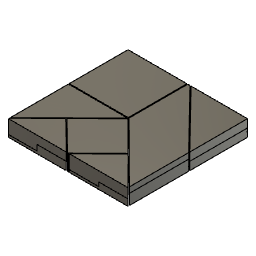
3D Puzzle Pieces v8 (Autodesk Fusion 360 design; units mm, degrees)
Autodesk Fusion 360 part; units mm, degrees
box "BoxPrimitive1" add length 300 width 300 height 18 placed x (0, 0, -1) y (-1, 0, 0) z (0, 1, 0) at (300, 0, 0) makes body 1 in component "CNC Safe Box v6"
sketch "Sketch3" plane through (0, 0, 0) normal (0, 0, 1) x (1, 0, 0) in component "CNC Safe Box v6"
  line L0 (0, 18) -> (0, 0)
  line L1 (0, 0) -> (300, 0)
  line L2 (300, 0) -> (300, 18)
  line L3 (300, 18) -> (0, 18)
  line L4 (42.8571, 18) -> (85.7143, 18)
  line L5 (85.7143, 18) -> (85.7143, 0)
  line L6 (85.7143, 0) -> (42.8571, 0)
  line L7 (42.8571, 0) -> (42.8571, 18)
  dimension "d20" = 42.8571
  dimension "d21" = 18
  dimension "d22" = 42.8571
  constraint horizontal L4
  constraint vertical L5
  constraint horizontal L6
  constraint vertical L7
  constraint coincident L3 L4.start
  measures "d20" distance of L4.start L4.end
  measures "d21" distance of L4.start L6.end
  measures "d22" distance of L0.start L4.start
extrude "Extrude1" cut sketch "Sketch3" against normal blind 18 contours L1 L3 L4 L5 L6 L7 bodies 1 in component "CNC Safe Box v6"
pattern_linear "R-Pattern1" count 3 spacing 85.7143 along (1, 0, 0) of 3 faces at (42.8571, 6, -6) (57.1429, 12, -18) (85.7143, 12, -6) on bodies 1 in component "CNC Safe Box v6"
sketch "Sketch4" plane through (0, 0, 0) normal (-1, 0, 0) x (0, 0, 1) in component "CNC Safe Box v6"
  line L0 (-300, 18) -> (-300, 0)
  line L1 (-300, 0) -> (0, 0)
  line L2 (0, 0) -> (0, 18)
  line L3 (0, 18) -> (-300, 18)
  line L4 (-42.8571, 18) -> (-85.7143, 18)
  line L5 (-85.7143, 18) -> (-85.7143, 0)
  line L6 (-85.7143, 0) -> (-42.8571, 0)
  line L7 (-42.8571, 0) -> (-42.8571, 18)
  dimension "d29" = 42.8571
  dimension "d30" = 18
  dimension "d31" = 42.8571
  constraint horizontal L4
  constraint vertical L5
  constraint horizontal L6
  constraint vertical L7
  constraint coincident L3 L4.start
  measures "d29" distance of L4.start L4.end
  measures "d30" distance of L4.start L6.end
  measures "d31" distance of L2.end L4.start
extrude "Extrude2" cut sketch "Sketch4" against normal blind 18 contours L1 L3 L4 L5 L6 L7 bodies 1 in component "CNC Safe Box v6"
pattern_linear "R-Pattern2" count 3 spacing 85.7143 along (0, 0, -1) of 3 faces at (6, 6, -42.8571) (18, 12, -71.4286) (6, 12, -85.7143) on bodies 1 in component "CNC Safe Box v6"
sketch "Sketch5" plane through (0, 0, 0) normal (0, 0, 1) x (1, 0, 0) in component "CNC Safe Box v6"
  line L0 (0, 0) -> (300, 0)
  line L1 (300, 0) -> (300, 300)
  line L2 (300, 300) -> (0, 300)
  line L3 (0, 300) -> (0, 0)
  dimension "d38" = 300
  dimension "d39" = 300
  constraint horizontal L0
  constraint vertical L1
  constraint horizontal L2
  constraint vertical L3
  constraint coincident L0.start L3.end
  measures "d38" distance of L0.start L0.end
  measures "d39" distance of L0.start L2.end
extrude "Extrude3" add sketch "Sketch5" against normal blind 18 separate body makes body 2 in component "CNC Safe Box v6"
combine "Combine1" operation cut target body 2 tool bodies 1 keep tools in component "CNC Safe Box v6"
sketch "Sketch6" plane through (0, 0, 0) normal (-1, 0, 0) x (0, 0, 1) in component "CNC Safe Box v6"
  line L0 (-18, 18) -> (0, 18)
  line L1 (0, 18) -> (0, 300)
  line L2 (0, 300) -> (-18, 300)
  line L3 (-18, 300) -> (-18, 18)
  line L4 (-18, 60.8571) -> (0, 60.8571)
  line L5 (0, 60.8571) -> (0, 103.7143)
  line L6 (0, 103.7143) -> (-18, 103.7143)
  line L7 (-18, 103.7143) -> (-18, 60.8571)
  dimension "d42" = 18
  dimension "d43" = 42.8571
  dimension "d44" = 42.8571
  constraint horizontal L4
  constraint vertical L5
  constraint horizontal L6
  constraint vertical L7
  constraint coincident L3 L4.start
  measures "d42" distance of L4.start L4.end
  measures "d43" distance of L4.start L6.end
  measures "d44" distance of L0.start L4.start
extrude "Extrude4" cut sketch "Sketch6" against normal blind 18 contours L1 L3 L4 L5 L6 L7 bodies 2 in component "CNC Safe Box v6"
pattern_linear "R-Pattern3" count 3 spacing 85.7143 along (0, 1, 0) of 3 faces at (6, 60.8571, -12) (18, 89.4286, -12) (6, 103.7143, -6) on bodies 2 in component "CNC Safe Box v6"
sketch "Sketch7" plane through (0, 0, 0) normal (1, 0, 0) x (0, 0, -1) in component "CNC Safe Box v6"
  line L0 (0, 0) -> (300, 0)
  line L1 (300, 0) -> (300, 300)
  line L2 (300, 300) -> (0, 300)
  line L3 (0, 300) -> (0, 0)
  dimension "d54" = 300
  dimension "d55" = 300
  constraint horizontal L0
  constraint vertical L1
  constraint horizontal L2
  constraint vertical L3
  constraint coincident L0.start L3.end
  measures "d54" distance of L0.start L0.end
  measures "d55" distance of L0.start L2.end
extrude "Extrude6" add sketch "Sketch7" along normal blind 18 separate body makes body 3 in component "CNC Safe Box v6"
combine "Combine3" operation cut target body 3 tool bodies 2 1 keep tools in component "CNC Safe Box v6"
extrude "Extrude7" add 1 faces at (18, 169.1429, -163.1429) along direction (-1, 0, 0) blind 18 from surface at -282 separate body on bodies 3 makes body 4 in component "CNC Safe Box v6"
combine "Combine4" operation cut target body 1 tool bodies 4 keep tools in component "CNC Safe Box v6"
combine "Combine5" operation cut target body 2 tool bodies 4 keep tools in component "CNC Safe Box v6"
sketch "Sketch8" plane through (0, 0, 0) normal (0, 0, 1) x (1, 0, 0) in component "CNC Safe Box v6"
  line L0 (282, 275.1429) -> (300, 275.1429)
  line L1 (300, 275.1429) -> (300, 300)
  line L2 (300, 300) -> (0, 300)
  line L3 (0, 300) -> (0, 275.1429)
  line L4 (0, 275.1429) -> (18, 275.1429)
  line L5 (18, 275.1429) -> (18, 232.2857)
  line L6 (18, 232.2857) -> (0, 232.2857)
  line L7 (0, 232.2857) -> (0, 189.4286)
  line L8 (0, 189.4286) -> (18, 189.4286)
  line L9 (18, 189.4286) -> (18, 146.5714)
  line L10 (18, 146.5714) -> (0, 146.5714)
  line L11 (0, 146.5714) -> (0, 103.7143)
  line L12 (0, 103.7143) -> (18, 103.7143)
  line L13 (18, 103.7143) -> (18, 60.8571)
  line L14 (18, 60.8571) -> (0, 60.8571)
  line L15 (0, 60.8571) -> (0, 18)
  line L16 (0, 18) -> (42.8571, 18)
  line L17 (42.8571, 18) -> (42.8571, 0)
  line L18 (42.8571, 0) -> (85.7143, 0)
  line L19 (85.7143, 0) -> (85.7143, 18)
  line L20 (85.7143, 18) -> (128.5714, 18)
  line L21 (128.5714, 18) -> (128.5714, 0)
  line L22 (128.5714, 0) -> (171.4286, 0)
  line L23 (171.4286, 0) -> (171.4286, 18)
  line L24 (171.4286, 18) -> (214.2857, 18)
  line L25 (214.2857, 18) -> (214.2857, 0)
  line L26 (214.2857, 0) -> (257.1429, 0)
  line L27 (257.1429, 0) -> (257.1429, 18)
  line L28 (257.1429, 18) -> (300, 18)
  line L29 (300, 18) -> (300, 60.8571)
  line L30 (300, 60.8571) -> (282, 60.8571)
  line L31 (282, 60.8571) -> (282, 103.7143)
  line L32 (282, 103.7143) -> (300, 103.7143)
  line L33 (300, 103.7143) -> (300, 146.5714)
  line L34 (300, 146.5714) -> (282, 146.5714)
  line L35 (282, 146.5714) -> (282, 189.4286)
  line L36 (282, 189.4286) -> (300, 189.4286)
  line L37 (300, 189.4286) -> (300, 232.2857)
  line L38 (300, 232.2857) -> (282, 232.2857)
  line L39 (282, 232.2857) -> (282, 275.1429)
  circle A0 centre (269, 300) radius 13
  line L40 (300, 300) -> (240, 300)
  line L41 (240, 300) -> (240, 320)
  line L42 (240, 320) -> (300, 320)
  line L43 (300, 320) -> (300, 300)
  dimension "d61" = 26
  dimension "d62" = 31
  dimension "d66" = 60
  dimension "d67" = 20
  constraint coincident L2 A0.centre
  constraint horizontal L40
  constraint vertical L41
  constraint horizontal L42
  constraint vertical L43
  constraint coincident L1.end L2.start
  measures "d61" diameter of A0
  measures "d62" distance of L1.end A0.centre
  measures "d66" distance of L41.end L42.end
  measures "d67" distance of L40.end L41.end
extrude "Extrude8" add sketch "Sketch8" against normal blind 18 contours L2 A0 L40 L41 L42 L43 bodies 2 in component "CNC Safe Box v6"
extrude "Extrude9" cut sketch "Sketch8" against normal blind 18 contours L2 A0 L40 picked at (269.3238, 295.6788) bodies 2 in component "CNC Safe Box v6"
extrude "Extrude10" add 1 faces at (142.8571, 103.7143, -18) along direction (0, 0, 1) blind 18 from surface at -282 separate body on bodies 2 makes body 5 in component "CNC Safe Box v6"
combine "Combine7" operation cut target body 3 tool bodies 5 keep tools in component "CNC Safe Box v6"
combine "Combine8" operation cut target body 1 tool bodies 5 keep tools in component "CNC Safe Box v6"
combine "Combine9" operation cut target body 4 tool bodies 5 keep tools in component "CNC Safe Box v6"
sketch "Sketch9" plane through (0, 300, 0) normal (0, 1, 0) x (-1, 0, 0) in component "CNC Safe Box v6"
  line L0 (-18, -282) -> (0, -282)
  line L1 (0, -282) -> (0, -18)
  line L2 (0, -18) -> (-18, -18)
  line L3 (-18, -18) -> (-18, -282)
  line L4 (-18, -18) -> (-278, -18)
  line L5 (-278, -18) -> (-278, -282)
  line L6 (-278, -282) -> (-18, -282)
  line L7 (-18, -282) -> (-18, -18)
  line L8 (-278, -20.5856) -> (-277, -20.5856) construction
  line L9 (-277, -20.5856) -> (-260, -20.5856) construction
  line L10 (-268.5, -20.5856) -> (-268.5, -18)
  dimension "d75" = 260
  dimension "d76" = 264
  dimension "d77" = 1
  constraint horizontal L4
  constraint vertical L5
  constraint horizontal L6
  constraint vertical L7
  constraint coincident L2.end L3.start
  constraint coincident L5 L8.start
  constraint perpendicular L5 L8
  constraint parallel L8 L9
  constraint midpoint L9 L10.start
  constraint coincident L4 L10.end
  constraint perpendicular L4 L10
  measures "d75" distance of L2.end L4.end
  measures "d76" distance of L2.end L0.start
  measures "d77" distance of L8.start L8.end
extrude "Extrude11" add sketch "Sketch9" along normal mid plane 18 separate body contours L3 L4 L5 L6 L7 makes body 6 in component "CNC Safe Box v6"
extrude "Extrude13" add 2 faces at (80, 300, -294) (160, 300, -6) along direction (0, 1, 0) blind 9 on bodies 2 5 bodies 5 2 in component "CNC Safe Box v6"
extrude "Extrude14" add 2 faces at (6, 300, -194) (294, 300, -194) along direction (0, 1, 0) blind 9 on bodies 3 4 bodies 3 4 in component "CNC Safe Box v6"
sketch "Sketch10" plane through (0, 0, -18) normal (0, 0, 1) x (1, 0, 0) in component "CNC Safe Box v6"
  line L0 (278, 291) -> (278, 309)
  line L1 (278, 309) -> (18, 309)
  line L2 (18, 309) -> (18, 291)
  line L3 (18, 291) -> (278, 291)
  line L4 (278, 309) -> (260, 309)
  line L5 (260, 309) -> (260, 291)
  line L6 (260, 291) -> (278, 291)
  line L7 (278, 291) -> (278, 309)
  dimension "d86" = 18
  dimension "d87" = 18
  constraint horizontal L4
  constraint vertical L5
  constraint horizontal L6
  constraint vertical L7
  constraint coincident L0.end L1.start
  measures "d86" distance of L0.end L4.end
  measures "d87" distance of L0.end L0.start
extrude "Extrude15" add sketch "Sketch10" along normal blind 18 contours L0 L1 L3 L4 L5 L6 L7 bodies 6 in component "CNC Safe Box v6"
sketch "Sketch11" plane through (0, 0, -282) normal (0, 0, -1) x (-1, 0, 0) in component "CNC Safe Box v6"
  line L0 (-18, 291) -> (-18, 309)
  line L1 (-18, 309) -> (-278, 309)
  line L2 (-278, 309) -> (-278, 291)
  line L3 (-278, 291) -> (-18, 291)
  line L4 (-278, 309) -> (-260, 309)
  line L5 (-260, 309) -> (-260, 291)
  line L6 (-260, 291) -> (-278, 291)
  line L7 (-278, 291) -> (-278, 309)
  dimension "d90" = 18
  dimension "d91" = 18
  constraint horizontal L4
  constraint vertical L5
  constraint horizontal L6
  constraint vertical L7
  constraint coincident L1.end L2.start
  measures "d90" distance of L1.end L4.end
  measures "d91" distance of L1.end L2.end
extrude "Extrude16" add sketch "Sketch11" along normal blind 18 contours L1 L2 L3 L4 L5 L6 L7 bodies 6 in component "CNC Safe Box v6"
sketch "Sketch12" plane through (18, 0, 0) normal (-1, 0, 0) x (0, 0, 1) in component "CNC Safe Box v6"
  line L0 (-18, 291) -> (-18, 309)
  line L1 (-18, 309) -> (-282, 309)
  line L2 (-282, 309) -> (-282, 291)
  line L3 (-282, 291) -> (-18, 291)
  line L4 (-75, 309) -> (-225, 309)
  line L5 (-225, 309) -> (-225, 291)
  line L6 (-225, 291) -> (-75, 291)
  line L7 (-75, 291) -> (-75, 309)
  line L8 (-75, 309) -> (-225, 291) construction
  line L9 (-225, 309) -> (-75, 291) construction
  point P0 (-150, 300)
  dimension "d94" = 150
  dimension "d95" = 18
  constraint horizontal L4
  constraint perpendicular L4 L5
  constraint parallel L4 L6
  constraint parallel L5 L7
  constraint coincident L8 P0
  constraint coincident L9 P0
  measures "d94" distance of L5.end L6.end
  measures "d95" distance of L4.end L5.end
extrude "Extrude17" add sketch "Sketch12" along normal blind 50 contours L0 L1 L3 L7 | L1 L2 L3 L5 bodies 6 in component "CNC Safe Box v6"
extrude "Extrude18" add 1 faces at (18, 297, -125) along direction (1, 0, 0) blind 18 from surface at -50 on bodies 6 bodies 6 in component "CNC Safe Box v6"
combine "Combine10" operation cut target body 3 tool bodies 6 keep tools in component "CNC Safe Box v6"
fillet "Fillet1" radius 10 4 edges at (-14, 300, -225) (-14, 300, -75) (-32, 300, -18) (-32, 300, -282) on bodies 6 in component "CNC Safe Box v6"
fillet "Fillet2" radius 4 4 edges at (300, 320, -9) (240, 320, -9) (300, 320, -291) (240, 320, -291) on bodies 2 5 in component "CNC Safe Box v6"
sketch "Sketch13" plane through (0, 309, 0) normal (0, 1, 0) x (-1, 0, 0) in component "CNC Safe Box v6"
  arc A0 (22, -282) -> (32, -272) centre (22, -272) ccw
  line L0 (32, -272) -> (32, -28)
  arc A1 (32, -28) -> (22, -18) centre (22, -28) ccw
  line L1 (22, -18) -> (-260, -18)
  line L2 (-260, -18) -> (-260, 0)
  line L3 (-260, 0) -> (-278, 0)
  line L4 (-278, 0) -> (-278, -300)
  line L5 (-278, -300) -> (-260, -300)
  line L6 (-260, -300) -> (-260, -282)
  line L7 (-260, -282) -> (22, -282)
  line L8 (4, -225) -> (-18, -225)
  line L9 (-18, -225) -> (-18, -75)
  line L10 (-18, -75) -> (4, -75)
  arc A2 (14, -85) -> (4, -75) centre (4, -85) ccw
  line L11 (14, -85) -> (14, -215)
  arc A3 (4, -225) -> (14, -215) centre (4, -215) ccw
  line L12 (-226.3405, -74.4217) -> (-76.3405, -74.4217)
  line L13 (-76.3405, -74.4217) -> (-76.3405, -224.4217)
  line L14 (-76.3405, -224.4217) -> (-226.3405, -224.4217)
  line L15 (-226.3405, -224.4217) -> (-226.3405, -74.4217)
  line L16 (-226.3405, -74.4217) -> (-76.3405, -224.4217) construction
  line L17 (-76.3405, -74.4217) -> (-226.3405, -224.4217) construction
  line L18 (-68.3405, -66.4217) -> (-68.3405, -232.4217)
  line L19 (-68.3405, -232.4217) -> (-234.3405, -232.4217)
  line L20 (-234.3405, -232.4217) -> (-234.3405, -66.4217)
  line L21 (-234.3405, -66.4217) -> (-68.3405, -66.4217)
  line L22 (-55.3405, -53.4217) -> (-55.3405, -245.4217)
  line L23 (-55.3405, -245.4217) -> (-247.3405, -245.4217)
  line L24 (-247.3405, -245.4217) -> (-247.3405, -53.4217)
  line L25 (-247.3405, -53.4217) -> (-55.3405, -53.4217)
  circle A4 centre (-242, -240) radius 3.5
  point P0 (-151.3405, -149.4217)
  dimension "d108" = 150
  dimension "d109" = 150
  dimension "d113" = -8
  dimension "d121" = 7
  constraint horizontal L12
  constraint perpendicular L12 L13
  constraint parallel L12 L14
  constraint parallel L13 L15
  constraint coincident L16 P0
  constraint coincident L17 P0
  measures "d108" distance of L13.end L14.end
  measures "d109" distance of L12.end L13.end
  measures "d121" diameter of A4
extrude "Extrude19" cut sketch "Sketch13" against normal blind 15 contours L12 L13 L14 L15 bodies 6 in component "CNC Safe Box v6"
extrude "Extrude20" cut sketch "Sketch13" against normal blind 5 contours L22 L23 L24 L25 | A4 bodies 6 in component "CNC Safe Box v6"
extrude "Extrude21" cut sketch "Sketch13" against normal blind 18 contours A4 bodies 6 in component "CNC Safe Box v6"
sketch "Sketch1" plane through (0, 294, 0) normal (0, 1, 0) x (-1, 0, 0)
  line L0 (-226.3405, -224.4217) -> (-76.3405, -224.4217)
  line L1 (-76.3405, -224.4217) -> (-76.3405, -74.4217)
  line L2 (-76.3405, -74.4217) -> (-226.3405, -74.4217)
  line L3 (-226.3405, -74.4217) -> (-226.3405, -224.4217)
  line L4 (-77.3405, -223.4217) -> (-77.3405, -75.4217) construction
  line L5 (-77.3405, -75.4217) -> (-225.3405, -75.4217) construction
  line L6 (-225.3405, -75.4217) -> (-225.3405, -223.4217) construction
  line L7 (-225.3405, -223.4217) -> (-77.3405, -223.4217) construction
  line L8 (-150.3531, -150.7211) -> (-77.3405, -150.7211)
  line L9 (-77.3405, -150.7211) -> (-77.3405, -223.4217)
  line L10 (-77.3405, -223.4217) -> (-150.3531, -223.4217)
  line L11 (-150.3531, -223.4217) -> (-150.3531, -150.7211)
  line L12 (-150.3531, -213.4508) -> (-151.3531, -213.4508) construction
  line L13 (-150.3531, -182.8688) -> (-151.3531, -182.8688) construction
  line L14 (-150.3531, -156.3222) -> (-151.3531, -156.3222) construction
  line L15 (-151.3531, -150.7211) -> (-151.3405, -223.4217)
  line L16 (-151.3405, -223.4217) -> (-154.0836, -223.4222)
  line L17 (-154.0836, -223.4222) -> (-225.3405, -150.5544)
  line L18 (-225.3405, -150.5544) -> (-225.3405, -77.1999)
  line L19 (-151.3531, -150.7211) -> (-225.3405, -77.1999)
  line L20 (-175.6421, -201.3763) -> (-176.348, -202.0846) construction
  line L21 (-197.2035, -179.3275) -> (-197.9184, -180.0266) construction
  line L22 (-155.4827, -223.4217) -> (-225.3405, -223.4217)
  line L23 (-225.3405, -223.4217) -> (-225.3405, -152)
  line L24 (-159.0347, -143.088) -> (-158.3298, -142.3786) construction
  line L25 (-173.2488, -128.9634) -> (-172.544, -128.2541) construction
  line L26 (-196.8551, -105.5059) -> (-196.1502, -104.7965) construction
  line L27 (-216.7935, -85.693) -> (-216.0887, -84.9837) construction
  line L28 (-225.3405, -75.4217) -> (-196.1502, -104.7965)
  line L29 (-225.3405, -75.4217) -> (-152.6238, -75.4217)
  line L30 (-196.1502, -104.7965) -> (-158.3298, -142.3786)
  line L31 (-152.6238, -75.4217) -> (-189.3503, -111.5536)
  line L32 (-83.8807, -150.7211) -> (-83.8807, -149.7211) construction
  line L33 (-106.7755, -150.7211) -> (-106.7755, -149.7211) construction
  line L34 (-123.9792, -150.7211) -> (-123.9792, -149.7211) construction
  line L35 (-142.4493, -150.7211) -> (-142.4493, -149.7211) construction
  line L36 (-77.3405, -149.7211) -> (-150.3531, -149.7211)
  line L37 (-150.3531, -149.7211) -> (-77.3405, -77.654)
  line L38 (-77.3405, -77.654) -> (-77.3405, -149.7211)
  line L39 (-144.7949, -144.2349) -> (-145.4974, -143.5232) construction
  line L40 (-136.556, -136.1026) -> (-137.2585, -135.3909) construction
  line L41 (-125.9749, -125.6586) -> (-126.6774, -124.9469) construction
  line L42 (-112.4456, -112.3045) -> (-113.1481, -111.5928) construction
  line L43 (-102.2409, -102.232) -> (-102.9434, -101.5203) construction
  line L44 (-87.6709, -87.8506) -> (-88.3734, -87.1389) construction
  line L45 (-145.4974, -143.5232) -> (-151.3573, -149.3072)
  line L46 (-151.3573, -149.3072) -> (-158.3298, -142.3786)
  line L47 (-145.4974, -143.5232) -> (-88.3734, -87.1389)
  line L48 (-88.3734, -87.1389) -> (-77.3405, -76.2489)
  line L49 (-77.3405, -76.2489) -> (-77.3405, -75.4217)
  line L50 (-77.3405, -75.4217) -> (-149, -75.4217)
  line L51 (-112.6451, -111.0963) -> (-149, -75.4217)
  line L52 (-114.6172, -109.161) -> (-115.3176, -109.8748) construction
  line L53 (-123.6623, -100.2852) -> (-124.3627, -100.999) construction
  line L54 (-135.3985, -88.7686) -> (-136.0989, -89.4824) construction
  line L55 (-154.2294, -77.0013) -> (-153.5281, -77.7142) construction
  line L56 (-167.1927, -89.7548) -> (-166.4914, -90.4676) construction
  line L57 (-179.8404, -102.1977) -> (-179.1391, -102.9105) construction
  line L58 (-147.0492, -77.336) -> (-147.7496, -78.0497) construction
  line L59 (-147.7496, -78.0497) -> (-150.4278, -75.4217)
  line L60 (-150.4278, -75.4217) -> (-151.1979, -75.4217)
  line L61 (-147.7496, -78.0497) -> (-113.3568, -111.7988)
  circle A0 centre (-113.8468, -187.0714) radius 4.1
  line L62 (-101.859, -150.7211) -> (-101.859, -223.4217)
  line L63 (-125.481, -150.7211) -> (-125.481, -223.4217)
  line L64 (-77.3405, -149.7211) -> (-113.8468, -113.6876)
  line L65 (-133.1739, -131.3593) -> (-170.0039, -93.9232)
  line L66 (-189.3503, -111.5536) -> (-188.9821, -75.4217)
  circle A1 centre (-100, -85) radius 4.1
  line L67 (-112.6451, -111.0963) -> (-112.6316, -75.4217)
  line L68 (-151.3531, -150.7211) -> (-225.3405, -150.5544)
  line L69 (-225.3405, -152) -> (-155.4827, -223.4217)
  line L70 (-225.3405, -223.4217) -> (-189.6384, -188.5014)
  line L71 (-151.1979, -75.4217) -> (-188.6409, -112.2585)
  dimension "d1" = -1
  dimension "d2" = 1
  dimension "d3" = 1
  dimension "d4" = 1
  dimension "d5" = 1
  dimension "d6" = 1
  dimension "d8" = 1
  dimension "d9" = 1
  dimension "d10" = 1
  dimension "d11" = 1
  dimension "d13" = 1
  dimension "d14" = 1
  dimension "d51" = 1
  dimension "d52" = 1
  dimension "d53" = 1
  dimension "d63" = 1
  dimension "d64" = 1
  dimension "d65" = 1
  dimension "d80" = 1
  dimension "d81" = 1
  dimension "d102" = 1
  dimension "d103" = 1
  dimension "d110" = 1
  dimension "d112" = 1
  dimension "d114" = 1
  dimension "d118" = 1
  dimension "d124" = 1
  dimension "d127" = 8.2
  dimension "d129" = 8.2
  constraint horizontal L8
  constraint vertical L9
  constraint horizontal L10
  constraint vertical L11
  constraint coincident L11 L12.start
  constraint perpendicular L11 L12
  constraint coincident L11 L13.start
  constraint perpendicular L11 L13
  constraint coincident L11 L14.start
  constraint perpendicular L11 L14
  constraint midpoint L7 L15.end
  constraint perpendicular L15 L16
  constraint coincident L6 L17.end
  constraint coincident L6 L18.end
  constraint perpendicular L5 L18
  constraint coincident L17 L20.start
  constraint coincident L17 L21.start
  constraint perpendicular L17 L21
  constraint coincident L7 L22.start
  constraint coincident L6 L23.end
  constraint perpendicular L7 L23
  constraint coincident L19 L24.start
  constraint perpendicular L19 L24
  constraint coincident L19 L25.start
  constraint perpendicular L19 L25
  constraint coincident L19 L26.start
  constraint perpendicular L19 L26
  constraint coincident L19 L27.start
  constraint perpendicular L19 L27
  constraint coincident L5 L29.end
  constraint coincident L30 L31.end
  constraint coincident L8 L32.start
  constraint perpendicular L8 L32
  constraint coincident L8 L33.start
  constraint perpendicular L8 L33
  constraint coincident L8 L34.start
  constraint perpendicular L8 L34
  constraint coincident L8 L35.start
  constraint perpendicular L8 L35
  constraint coincident L4 L36.start
  constraint perpendicular L11 L36
  constraint coincident L4 L37.end
  constraint coincident L37 L39.start
  constraint perpendicular L37 L39
  constraint coincident L37 L40.start
  constraint perpendicular L37 L40
  constraint coincident L37 L41.start
  constraint perpendicular L37 L41
  constraint coincident L37 L42.start
  constraint perpendicular L37 L42
  constraint coincident L37 L43.start
  constraint perpendicular L37 L43
  constraint coincident L37 L44.start
  constraint perpendicular L37 L44
  constraint perpendicular L39 L45
  constraint perpendicular L24 L46
  constraint coincident L4 L48.end
  constraint perpendicular L44 L48
  constraint coincident L5 L50.end
  constraint perpendicular L49 L50
  constraint coincident L47 L51.start
  constraint coincident L51 L52.start
  constraint perpendicular L51 L52
  constraint coincident L51 L53.start
  constraint perpendicular L51 L53
  constraint coincident L51 L54.start
  constraint perpendicular L51 L54
  constraint coincident L31 L55.start
  constraint perpendicular L31 L55
  constraint coincident L31 L56.start
  constraint perpendicular L31 L56
  constraint coincident L31 L57.start
  constraint perpendicular L31 L57
  constraint coincident L51 L58.start
  constraint perpendicular L51 L58
  constraint coincident L5 L60.end
  constraint coincident L5 L59.end
  constraint perpendicular L58 L59
  constraint coincident L47 L61.end
  constraint perpendicular L58 L61
  constraint vertical L62
  constraint coincident L8 L62.start
  constraint coincident L10 L62.end
  constraint vertical L63
  constraint coincident L8 L63.start
  constraint coincident L10 L63.end
  constraint midpoint L37 L64.end
  constraint coincident L47 L65.start
  constraint midpoint L29 L66.end
  constraint coincident L5 L67.end
  constraint coincident L69 L70.end
  constraint perpendicular L69 L70
  constraint coincident L30 L71.end
  constraint perpendicular L57 L71
  measures "d2" distance of L12.start L12.end
  measures "d3" distance of L13.start L13.end
  measures "d4" distance of L14.start L14.end
  measures "d5" distance of L20.start L20.end
  measures "d6" distance of L21.start L21.end
  measures "d8" distance of L24.start L24.end
  measures "d9" distance of L25.start L25.end
  measures "d10" distance of L26.start L26.end
  measures "d11" distance of L27.start L27.end
  measures "d13" distance of L32.start L32.end
  measures "d14" distance of L33.start L33.end
  measures "d51" distance of L34.start L34.end
  measures "d52" distance of L35.start L35.end
  measures "d53" distance of L39.start L39.end
  measures "d63" distance of L40.start L40.end
  measures "d64" distance of L41.start L41.end
  measures "d65" distance of L42.start L42.end
  measures "d80" distance of L43.start L43.end
  measures "d81" distance of L44.start L44.end
  measures "d102" distance of L52.start L52.end
  measures "d103" distance of L53.start L53.end
  measures "d110" distance of L54.start L54.end
  measures "d112" distance of L55.start L55.end
  measures "d114" distance of L56.start L56.end
  measures "d118" distance of L57.start L57.end
  measures "d124" distance of L58.start L58.end
  measures "d127" diameter of A0
  measures "d129" diameter of A1
extrude "Extrude1'" add sketch "Sketch1" along normal blind 12 separate body contours L8 L10 L11 L63 | L8 L9 L10 L62 makes body 7 at (93.6862, 294, -174.9547) makes body 8 at (142.0624, 294, -174.9547)
extrude "Extrude2'" add sketch "Sketch1" along normal blind 3 contours L8 L10 L62 L63 | A0 bodies 7 8
extrude "Extrude4'" add 1 faces at (126.0156, 294, -174.9547) along direction (0, 1, 0) blind 20 separate body on bodies 7 makes body 9
combine "Combine1'" operation cut target body 9 tool bodies 7 keep tools
extrude "Extrude5" cut sketch "Sketch1" along normal mid plane 2.8 from surface at 3 contours A0 bodies 7 9
extrude "Extrude6'" add sketch "Sketch1" along normal blind 6 separate body contours L22 L69 L70 | L23 L69 L70 makes body 10
extrude "Extrude7'" add sketch "Sketch1" along normal blind 10 contours L23 L69 L70 bodies 10
extrude "Extrude8'" add 1 faces at (202.0546, 294, -199.6145) along direction (0, 1, 0) blind 20 separate body on bodies 10 makes body 11
combine "Combine2" operation cut target body 11 tool bodies 10 keep tools
extrude "Extrude9'" add sketch "Sketch1" along normal blind 5 separate body contours L18 L19 L68 | L15 L16 L17 L68 makes body 12
extrude "Extrude10'" add sketch "Sketch1" along normal blind 13 contours L18 L19 L68 bodies 12
extrude "Extrude11'" add 1 faces at (176.9258, 294, -174.8992) along direction (0, 1, 0) blind 20 separate body on bodies 12 makes body 13
combine "Combine3'" operation cut target body 13 tool bodies 12 keep tools
extrude "Extrude12" add sketch "Sketch1" along normal blind 3 separate body contours L28 L29 L30 L66 | L29 L31 L66 makes body 14
extrude "Extrude13'" add sketch "Sketch1" along normal blind 8 contours L28 L29 L30 L66 bodies 14
extrude "Extrude14'" add 1 faces at (191.3715, 294, -85.2133) along direction (0, 1, 0) blind 20 separate body on bodies 14 makes body 15
combine "Combine4'" operation cut target body 15 tool bodies 14 keep tools
extrude "Extrude15'" add sketch "Sketch1" along normal blind 6 separate body contours L30 L45 L46 L47 L65 L71 | L47 L59 L60 L61 L65 L71 makes body 16
extrude "Extrude16'" add sketch "Sketch1" along normal blind 14 contours L47 L59 L60 L61 L65 L71 bodies 16
extrude "Extrude17'" add 1 faces at (138.3806, 294, -112.1759) along direction (0, 1, 0) blind 20 separate body on bodies 16 makes body 17
combine "Combine5'" operation cut target body 17 tool bodies 16 keep tools
extrude "Extrude18'" add sketch "Sketch1" along normal blind 3 separate body contours L47 L48 L49 L50 L67 | L50 L51 L67 | A1 makes body 18
extrude "Extrude19'" add sketch "Sketch1" along normal blind 10 contours L50 L51 L67 bodies 18
extrude "Extrude20'" add 1 faces at (112.9952, 294, -87.3132) along direction (0, 1, 0) blind 20 separate body on bodies 18 makes body 19
combine "Combine6" operation cut target body 19 tool bodies 18 keep tools
extrude "Extrude21'" cut sketch "Sketch1" along normal mid plane 2.8 from surface at 3 contours A1 bodies 18 19
extrude "Extrude22" add sketch "Sketch1" along normal blind 6 separate body contours L37 L38 L64 | L36 L37 L64 makes body 20
extrude "Extrude23" add sketch "Sketch1" along normal blind 10 contours L37 L38 L64 bodies 20
extrude "Extrude24" add 1 faces at (101.678, 294, -125.6988) along direction (0, 1, 0) blind 20 separate body on bodies 20 makes body 21
combine "Combine7'" operation cut target body 21 tool bodies 20 keep tools
component "CNC Safe Box v6" placed x (1, 0, 0) y (0, 1, 0) z (0, 0, 1) at (0, 0, 0)
hidden bodies 1 2 3 4 5 6
equation "Length = 300 mm"
equation "Width = 300 mm"
equation "Height = 300 mm"
equation "Thickness = 18 mm"
equation "LSTab = 3"
equation "WSTab = 3"
equation "HSTab = 3"
equation "LTabForm = Length / ( ( LSTab * 2 ) + 1 )"
equation "WTabForm = Width / ( ( WSTab * 2 ) + 1 )"
equation "HTabForm = Height / ( ( HSTab * 2 ) + 1 )"
equation "LPattForm = ( Length - ( LTabForm * 3 ) )"
equation "WPattForm = ( Width - ( WTabForm * 3 ) )"
equation "HPattForm = ( Height - ( HTabForm * 3 ) )"
equation "LidInnerHole = Thickness + 8 mm"
equation "d15 = Width"
equation "d16 = Length"
equation "d17 = Thickness"
equation "d20 = LTabForm"
equation "d21 = Thickness"
equation "d22 = LTabForm"
equation "d23 = -Thickness"
equation "d25 = LSTab"
equation "d27 = -LPattForm"
equation "d29 = WTabForm"
equation "d30 = Thickness"
equation "d31 = WTabForm"
equation "d32 = -Thickness"
equation "d34 = WSTab"
equation "d36 = -WPattForm"
equation "d38 = Length"
equation "d39 = Height"
equation "d40 = -Thickness"
equation "d42 = Thickness"
equation "d43 = HTabForm"
equation "d44 = HTabForm"
equation "d45 = -Thickness"
equation "d47 = HSTab"
equation "d49 = -HPattForm"
equation "d54 = Width"
equation "d55 = Height"
equation "d56 = Thickness"
equation "d59 = -Thickness"
equation "d61 = LidInnerHole"
equation "d62 = GapInnerHole"
equation "GapInnerHole = 31 mm"
equation "LHoleRec = 60 mm"
equation "HHoleRec = 20 mm"
equation "d66 = LHoleRec"
equation "d67 = HHoleRec"
equation "d68 = -Thickness"
equation "d70 = -Thickness"
equation "d73 = -Thickness"
equation "d78 = Thickness / 2"
equation "d86 = Thickness"
equation "d87 = Thickness"
equation "d88 = Thickness"
equation "d90 = Thickness"
equation "d91 = Thickness"
equation "d92 = Thickness"
equation "d95 = Thickness"
equation "Whandle = 50 mm"
equation "d97 = Whandle"
equation "d100 = -Thickness"
equation "FHandle = 10 mm"
equation "FHole = 4 mm"
equation "d105 = FHandle"
equation "d107 = FHole"
equation "d108 = WPuzzle"
equation "d109 = LPuzzle"
equation "LPuzzle = 150 mm"
equation "WPuzzle = 150 mm"
equation "DPuzzle = 15 mm"
equation "OLeds = 21 mm" comment "Offset for leds"
equation "d115 = -OLeds"
equation "d116 = -DPuzzle"
equation "DLeds = 5 mm"
equation "d119 = -DLeds"
equation "d122 = -Thickness"
equation "d2 = PuzzlePieceGap"
equation "d3 = PuzzlePieceGap"
equation "d4 = PuzzlePieceGap"
equation "d5 = PuzzlePieceGap"
equation "d6 = PuzzlePieceGap"
equation "d8 = PuzzlePieceGap"
equation "d9 = PuzzlePieceGap"
equation "d10 = PuzzlePieceGap"
equation "d11 = PuzzlePieceGap"
equation "d13 = PuzzlePieceGap"
equation "d14 = PuzzlePieceGap"
equation "d51 = PuzzlePieceGap"
equation "d52 = PuzzlePieceGap"
equation "d53 = PuzzlePieceGap"
equation "d63 = PuzzlePieceGap"
equation "d64 = PuzzlePieceGap"
equation "d65 = PuzzlePieceGap"
equation "d80 = PuzzlePieceGap"
equation "d81 = PuzzlePieceGap"
equation "PuzzlePieceGap = 1 mm"
equation "d102 = PuzzlePieceGap"
equation "d103 = PuzzlePieceGap"
equation "d110 = PuzzlePieceGap"
equation "d112 = PuzzlePieceGap"
equation "d114 = PuzzlePieceGap"
equation "d118 = PuzzlePieceGap"
equation "d124 = PuzzlePieceGap"
equation "DiameterMagnet = 8.2 mm"
equation "HMagnet = 2.8 mm"
equation "d127 = DiameterMagnet"
equation "d129 = DiameterMagnet"
equation "d139 = HMagnet / 2"
equation "d172 = HMagnet / 2"
named bodies: "MSquare1", "MSquare2", "TriangleT1", "TriangleT2", "Parallel1", "Parallel2", "2TriangleT1", "2TriangleT2", "2SquareS1", "2SquareS2", "MTriangleT1", "MTriangleT2", "4TriangleT1", "4TriangleT2"
